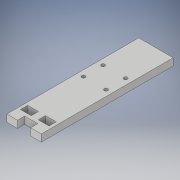
# Autodesk Inventor part: thumper-bumper-sidewall-v3
Saved by Autodesk Inventor 2017 (Build 210142000, 142)
## iProperties
Created: 2017-02-22
Part Number: thumper-bumper-sidewall-v3
Material: Generic
Document SubType Name: Modeling
Designer: John
Density: 1 g/cm^3
Appearance: Default
Author: John
Autodesk Inventor part; units mm, degrees
ref_plane "YZ Plane" through (0, 0, 0) normal (1, 0, 0) x (0, 1, 0)
ref_plane "XZ Plane" through (0, 0, 0) normal (0, 1, 0) x (-1, 0, 0)
ref_plane "XY Plane" through (0, 0, 0) normal (0, 0, 1) x (1, 0, 0)
sketch "Sketch1" plane through (0, 0, 0) normal (0, 1, 0) x (-1, 0, 0)
  line L0 (10.1226, -11.6524) -> (10.1226, 93.3476)
  line L1 (-18.8774, 93.3476) -> (-18.8774, -11.6524)
  line L2 (-18.8774, -11.6524) -> (-4.3774, -11.6524)
  line L3 (-4.3774, -11.6524) -> (-4.3774, 93.3476) construction
  line L4 (-18.8774, 40.8476) -> (-4.3774, 40.8476) construction
  line L5 (-18.8774, 93.3476) -> (10.1226, 93.3476)
  line L6 (-18.8774, 93.3476) -> (-9.8774, 93.3476)
  line L7 (-9.8774, 93.3476) -> (-9.8774, 99.3476)
  line L8 (-9.8774, 99.3476) -> (-18.8774, 99.3476)
  line L9 (-18.8774, 99.3476) -> (-18.8774, 93.3476)
  line L10 (10.1226, 93.3476) -> (1.1357, 93.3476)
  line L11 (1.1357, 93.3476) -> (1.1226, 99.3476)
  line L12 (1.1226, 99.3476) -> (10.1226, 99.3476)
  line L13 (10.1226, 99.3476) -> (10.1226, 93.3476)
  line L14 (-4.3774, 40.8476) -> (10.1226, 40.8476) construction
  line L15 (-4.3774, -11.6524) -> (10.1226, -11.6524)
  line L16 (-7.3774, 90.3476) -> (-16.3774, 90.3476)
  line L17 (-16.3774, 90.3476) -> (-16.3774, 84.3476)
  line L18 (-16.3774, 84.3476) -> (-7.3774, 84.3476)
  line L19 (-7.3774, 84.3476) -> (-7.3774, 90.3476)
  line L20 (-7.3774, 90.3476) -> (-16.3774, 84.3476) construction
  line L21 (-16.3774, 90.3476) -> (-7.3774, 84.3476) construction
  line L22 (-1.3774, 90.3476) -> (7.6226, 90.3476)
  line L23 (7.6226, 90.3476) -> (7.6226, 84.3476)
  line L24 (7.6226, 84.3476) -> (-1.3774, 84.3476)
  line L25 (-1.3774, 84.3476) -> (-1.3774, 90.3476)
  line L26 (-1.3774, 90.3476) -> (7.6226, 84.3476) construction
  line L27 (7.6226, 90.3476) -> (-1.3774, 84.3476) construction
  point P0 (-11.8774, 87.3476)
  point P1 (3.1226, 87.3476)
  dimension "d0" = 29
  dimension "d1" = 105
  dimension "d18" = 9
  dimension "d19" = 6
  dimension "d20" = 14.5
  dimension "d21" = 9
  dimension "d22" = 6
  dimension "d23" = 3
  dimension "d44" = 6
  constraints: 56 end point, 7 midpoint, 7 parallel, 5 equal length, 5 horizontal, 5 symmetric about line, 3 collinear, 2 perpendicular, 1 vertical
  measures "d0" distance of L1.start L0.end
  measures "d1" distance of L0.end L0.start
  measures "d18" distance of L8.end L7.end
  measures "d19" distance of L7.end L6.end
  measures "d20" distance between parallel lines of L3 L9
  measures "d21" distance of L18.end L17.end
  measures "d22" distance of L17.end L16.end
  measures "d23" distance between parallel lines of L5 L16
  measures "d44" distance between parallel lines of L19 L25
extrude "Extrusion1" add sketch "Sketch1" along normal blind 6
sketch "Sketch2" plane through (0, 6, 0) normal (0, 1, 0) x (1, 0, 0)
  circle A0 centre (-5.1253, -23.3476) radius 1.4986
  circle A1 centre (13.8747, -23.3476) radius 1.4986
  circle A2 centre (13.8747, -39.8476) radius 1.4985
  circle A3 centre (-5.1253, -39.8476) radius 1.4985
  line L0 (13.8747, -39.8476) -> (-5.1253, -39.8476) construction
  line L1 (-5.1253, -39.8476) -> (-5.1253, -23.3476) construction
  line L2 (-5.1253, -23.3476) -> (13.8747, -23.3476) construction
  line L3 (13.8747, -23.3476) -> (13.8747, -39.8476) construction
  line L4 (13.8747, -39.8476) -> (-5.1253, -23.3476) construction
  line L5 (13.8747, -23.3476) -> (-5.1253, -39.8476) construction
  line L6 (18.8774, 11.6524) -> (-10.1226, 11.6524) construction
  line L7 (4.3774, 11.6524) -> (4.3708, -93.3476) construction
  line L8 (-1.1357, -93.3476) -> (9.8774, -93.3476) construction
  point P0 (0, 0)
  point P1 (4.3747, -31.5976)
  dimension "d26" = 2.9972
  dimension "d28" = 2.9972
  dimension "d29" = 19
  dimension "d30" = 2.997
  dimension "d31" = 2.997
  dimension "d32" = 16.5
  dimension "d33" = 0
  dimension "d45" = 70
  constraints: 14 end point, 4 centre point, 3 midpoint, 3 perpendicular, 1 horizontal
  measures "d26" diameter of A0
  measures "d28" diameter of A1
  measures "d29" distance of L1.end L2.end
  measures "d30" diameter of A3
  measures "d31" diameter of A2
  measures "d32" distance of L2.end L0.start
  measures "d33" distance from line of L7 point (4.375, -31.598)
  measures "d45" distance from line of L8 L2.end
extrude "Extrusion2" cut sketch "Sketch2" against normal through all
body "Solid1"
